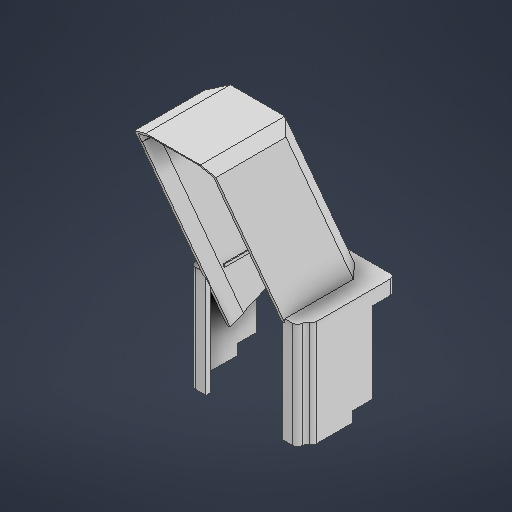
# Autodesk Inventor part: Event_Cover
Saved by Autodesk Inventor 2026 (Build 300175000, 175)
## iProperties
Created: 2025-07-07
Part Number: Event_Cover
Material: Generic
Document SubType Name: Modeling
Designer: Charl
Density: 1 g/cm^3
Appearance: Default
Author: Charl
Autodesk Inventor part; units mm, degrees
ref_plane "YZ Plane" through (0, 0, 0) normal (1, 0, 0) x (0, 1, 0)
ref_plane "XZ Plane" through (0, 0, 0) normal (0, 1, 0) x (-1, 0, 0)
sketch "Sketch1" plane through (0, 0, 0) normal (0, 1, 0) x (-1, 0, 0)
  line L0 (-58.5, -37.5625) -> (58.5, -37.5625)
  line L1 (58.5, -37.5625) -> (58.5, 37.5625)
  line L2 (58.5, 37.5625) -> (-58.5, 37.5625)
  line L3 (-58.5, 37.5625) -> (-58.5, -37.5625)
  line L4 (-58.5, -37.5625) -> (58.5, 37.5625) construction
  line L5 (58.5, -37.5625) -> (-58.5, 37.5625) construction
  line L6 (-61.5, 37.5625) -> (61.5, 37.5625)
  line L7 (61.5, 37.5625) -> (61.5, -40.5625)
  line L8 (61.5, -40.5625) -> (-61.5, -40.5625)
  line L9 (-61.5, -40.5625) -> (-61.5, 37.5625)
  line L10 (-38.5, 50.0625) -> (38.5, 50.0625)
  line L11 (38.5, 50.0625) -> (38.5, 25.0625)
  line L12 (38.5, 25.0625) -> (-38.5, 25.0625)
  line L13 (-38.5, 25.0625) -> (-38.5, 50.0625)
  line L14 (-38.5, 50.0625) -> (38.5, 25.0625) construction
  line L15 (38.5, 50.0625) -> (-38.5, 25.0625) construction
  line L16 (40, 37.5625) -> (40, 55.5625)
  line L17 (40, 55.5625) -> (55.75, 55.5625)
  line L18 (55.75, 55.5625) -> (55.75, 45.5625)
  line L19 (55.75, 45.5625) -> (61.5, 45.5625)
  line L20 (61.5, 45.5625) -> (61.5, 37.5625)
  line L21 (0, 358.9567) -> (0, -111.4305)
  line L22 (-40, 37.5625) -> (-40, 55.5625)
  line L23 (-40, 55.5625) -> (-55.75, 55.5625)
  line L24 (-55.75, 55.5625) -> (-55.75, 45.5625)
  line L25 (-55.75, 45.5625) -> (-61.5, 45.5625)
  line L26 (-61.5, 45.5625) -> (-61.5, 37.5625)
  circle A0 centre (0, 10.0625) radius 38.5
  line L27 (38.5, 25.0625) -> (-38.5, 25.0625)
  line L28 (-38.5, 25.0625) -> (-38.5, 10.0625)
  line L29 (-38.5, 10.0625) -> (38.5, 10.0625)
  line L30 (38.5, 10.0625) -> (38.5, 25.0625)
  point P0 (0, 0)
  point P1 (0, 37.5625)
  point P2 (-35.4577, 25.0625)
  point P3 (-38.5, 37.5625)
  point P4 (38.5, 37.5625)
  point P5 (35.4577, 25.0625)
  point P6 (38.5, 10.0625)
  dimension "d0" = 117
  dimension "d1" = 75.125
  dimension "d2" = 3
  dimension "d3" = 3
  dimension "d4" = 3
  dimension "d5" = 77
  dimension "d6" = 25
  dimension "d7" = 1.5
  dimension "d8" = 15.75
  dimension "d9" = 10
  dimension "d10" = 8
  dimension "d11" = 5.75
  dimension "d12" = 8
  dimension "d13" = 10
  dimension "d14" = 15.75
  dimension "d15" = 5.75
  dimension "d16" = 1.5
  dimension "d17" = 77
  dimension "d18" = 15
  dimension "d19" = 123
  dimension "d20" = 117
  dimension "d23" = 77
  constraints: 62 end point, 9 perpendicular, 8 parallel, 5 midpoint, 5 point on line, 5 symmetric about line, 3 horizontal, 1 centre point, 1 vertical
  measures "d0" distance of L2.end L1.end
  measures "d1" distance of L1.end L0.end
  measures "d2" distance between parallel lines of L1 L7
  measures "d3" distance between parallel lines of L9 L3
  measures "d4" distance between parallel lines of L8 L0
  measures "d5" distance of L11.end L12.end
  measures "d6" distance of L10.end L11.end
  measures "d7" distance from line of L11 L16.start
  measures "d8" distance of L16.end L17.end
  measures "d9" distance of L17.end L18.end
  measures "d10" distance of L19.end L6.end
  measures "d11" distance of L18.end L19.end
  measures "d12" distance of L26.start L6.start
  measures "d13" distance of L24.start L25.start
  measures "d14" distance of L23.start L24.start
  measures "d15" distance of L25.start L26.start
  measures "d16" distance between parallel lines of L13 L22
  measures "d17" diameter of A0
  measures "d18" distance from line of L12 A0.centre
  measures "d19" distance of L7.end L8.end
  measures "d20" distance of L0.start L0.end
  measures "d23" distance of L28.end L29.end
extrude "Extrusion2" add sketch "Sketch1" along normal blind 3 contours L3 L2 L13 L28 A0 L21 L0 | L0 L21 L8 L9 L6 L3 | L21 A0 L30 L11 L2 L1 L0 | L0 L1 L6 L7 L8 L21 | L6 L26 L25 L24 L23 L22 L2 | L2 L16 L17 L18 L19 L20 L6
sketch "Sketch3" plane through (0, 0, 0) normal (0, -1, 0) x (1, 0, 0)
  line L0 (-55.75, 55.5625) -> (-40, 55.5625) projected
  line L1 (-40, 55.5625) -> (-55.75, 55.5625)
  line L2 (-61.5, 45.5625) -> (-55.75, 45.5625) projected
  line L3 (-55.75, 55.5625) -> (-55.75, 45.5625)
  line L4 (-55.75, 45.5625) -> (-61.5, 45.5625)
  line L5 (-61.5, 45.5625) -> (-61.5, 20.5625)
  line L6 (-61.5, 20.5625) -> (-59.5, 20.5625)
  line L7 (-59.5, 20.5625) -> (-59.5, 43.5625)
  line L8 (-59.5, 43.5625) -> (-53.75, 43.5625)
  line L9 (-53.75, 43.5625) -> (-53.75, 50.5625)
  line L10 (-53.75, 50.5625) -> (-40, 50.5625)
  line L11 (-40, 55.5625) -> (-40, 37.5625) projected
  line L12 (-40, 55.5625) -> (-40, 50.5625)
  line L13 (55.75, 55.5625) -> (40, 55.5625)
  line L14 (40, 55.5625) -> (55.75, 55.5625)
  line L15 (61.5, 45.5625) -> (55.75, 45.5625)
  line L16 (55.75, 55.5625) -> (55.75, 45.5625)
  line L17 (55.75, 45.5625) -> (61.5, 45.5625)
  line L18 (61.5, 45.5625) -> (61.5, 20.5625)
  line L19 (61.5, 20.5625) -> (59.5, 20.5625)
  line L20 (59.5, 20.5625) -> (59.5, 43.5625)
  line L21 (59.5, 43.5625) -> (53.75, 43.5625)
  line L22 (53.75, 43.5625) -> (53.75, 50.5625)
  line L23 (53.75, 50.5625) -> (40, 50.5625)
  line L24 (40, 55.5625) -> (40, 37.5625)
  line L25 (40, 55.5625) -> (40, 50.5625)
  point P0 (0, 0)
  dimension "d31" = 5
  dimension "d32" = 2
  dimension "d33" = 2
  dimension "d34" = 25
  dimension "d35" = 2
  constraints: 46 end point, 7 perpendicular, 2 collinear, 2 point on line, 1 horizontal
  measures "d31" distance of L0.end L10.end
  measures "d32" distance between parallel lines of L3 L9
  measures "d33" distance between parallel lines of L2 L8
  measures "d34" distance between parallel lines of L6 L2
  measures "d35" distance between parallel lines of L5 L7
extrude "Extrusion3" add sketch "Sketch3" along normal blind 107.5
sketch "Sketch4" plane through (0, 0, 0) normal (0, -1, 0) x (1, 0, 0)
  line L0 (61.5, -40.5625) -> (-61.5, -40.5625)
  line L1 (61.5, -40.5625) -> (61.5, -16.5625)
  line L2 (61.5, -16.5625) -> (56, -16.5625)
  line L3 (56, -16.5625) -> (56, -37.5625)
  line L4 (56, -37.5625) -> (-56, -37.5625)
  line L5 (-56, -37.5625) -> (-56, -16.5625)
  line L6 (-56, -16.5625) -> (-61.5, -16.5625)
  line L7 (-61.5, -16.5625) -> (-61.5, -40.5625)
  line L8 (61.5, -17.0329) -> (61.5, 20.5625)
  line L9 (59.5, 43.5625) -> (59.5, 20.5625) projected
  line L10 (59.5, 20.5625) -> (59.5, -16.5625)
  line L11 (-61.5, 20.5625) -> (-59.5, 20.5625) projected
  line L12 (-59.5, 20.5625) -> (-59.5, -16.5625)
  line L13 (-61.5, -40.5625) -> (-61.5, 45.5625) projected
  line L14 (-61.5, 20.5625) -> (-61.5, -16.5625)
  line L15 (61.5, 20.5625) -> (61.5, 45.5625) projected
  line L16 (61.5, 20.5625) -> (59.5, 20.5625)
  line L17 (-59.5, 20.5625) -> (-61.5, 20.5625)
  point P0 (0, 0)
  dimension "d38" = 24
  dimension "d39" = 24
  dimension "d40" = 5.5
  dimension "d41" = 5.5
  dimension "d42" = 3
  dimension "d43" = 2
  dimension "d44" = 2
  constraints: 28 end point, 6 perpendicular, 4 point on line, 3 horizontal, 3 vertical, 1 collinear
  measures "d38" distance between parallel lines of L0 L6
  measures "d39" distance of L0.start L1.end
  measures "d40" distance of L1.end L2.end
  measures "d41" distance of L5.end L6.end
  measures "d42" distance between parallel lines of L0 L4
  measures "d43" distance between parallel lines of L8 L10
  measures "d44" distance between parallel lines of L13 L12
extrude "Extrusion4" add sketch "Sketch4" along normal blind 12
fillet "Fillet1" radius 5 16 edges at (-55.75, -52.25, 55.5625) (-55.75, -52.25, 45.5625) (-61.5, -52.25, 45.5625) (-61.5, -4.5, -40.5625) (61.5, -4.5, -40.5625) (55.75, -52.25, 45.5625) (55.75, -52.25, 55.5625) (61.5, -52.25, 45.5625) (53.75, -53.75, 50.5625) (59.5, -53.75, 43.5625) (53.75, -53.75, 43.5625) (-53.75, -53.75, 50.5625) (-53.75, -53.75, 43.5625) (-59.5, -53.75, 43.5625) (56, -6, -37.5625) (-56, -6, -37.5625)
chamfer "Chamfer1" distance 3.5 angle 45 2 edges at (56, -6, -16.5625) (-56, -6, -16.5625)
ref_plane "Work Plane1" through (-55.75, 3, 55.5625) normal (0, 0.9187912, 0.3947439) x (1, 0, 0)
sketch "Sketch5" plane through (-55.75, 3, 55.5625) normal (0, 0.9187912, 0.3947439) x (1, 0, 0)
  line L0 (16.25, 24.0537) -> (16.25, 75.6785)
  line L1 (16.25, 75.6785) -> (95.25, 75.6785)
  line L2 (95.25, 75.6785) -> (95.25, 24.0537)
  line L3 (55.75, 49.8661) -> (16.25, 75.6785) construction
  line L4 (55.75, 49.8661) -> (95.25, 75.6785) construction
  line L5 (13.25, 20.0537) -> (13.25, 79.6785)
  line L6 (13.25, 79.6785) -> (98.25, 79.6785)
  line L7 (98.25, 79.6785) -> (98.25, 20.0537)
  line L8 (55.75, 49.8661) -> (98.25, 79.6785) construction
  ellipse E0 centre (55.75, 40.6208) end of major axis (94.25, 40.6208) minor radius 35.3735 (94.25, 40.6208) -> (17.25, 40.6208) ccw projected
  ellipse E1 centre (55.75, 41.805) end of major axis (94.25, 41.805) minor radius 35.3735 (94.25, 41.805) -> (17.25, 41.805) ccw projected
  line L9 (5, 0) -> (15.75, 0) construction
  line L10 (-163.9514, 0) -> (184.7014, 0) construction
  line L11 (13.25, 20.0537) -> (13.25, -1.5)
  line L12 (13.25, -1.5) -> (16.75, -1.5)
  line L13 (16.75, -1.5) -> (16.75, 13.3942)
  line L14 (16.75, 13.3942) -> (16.25, 13.3942)
  line L15 (16.25, 13.3942) -> (16.25, 20.0537)
  line L16 (55.75, 49.8661) -> (13.25, 79.6785) construction
  line L17 (16.25, 24.0537) -> (16.25, 20.0537)
  line L18 (17.25, 15.354) -> (17.25, 40.6208) projected
  line L19 (55.75, 112.6041) -> (55.75, -12.8719)
  line L20 (55.75, 112.6041) -> (181.2261, 112.6041) construction
  line L21 (95.25, 24.0537) -> (95.25, 75.6785)
  line L22 (98.25, 20.0537) -> (98.25, 79.6785)
  line L23 (106.5, 0) -> (95.75, 0) construction
  line L24 (98.25, 20.0537) -> (98.25, -1.5)
  line L25 (98.25, -1.5) -> (94.75, -1.5)
  line L26 (94.75, -1.5) -> (94.75, 13.3942)
  line L27 (94.75, 13.3942) -> (95.25, 13.3942)
  line L28 (95.25, 13.3942) -> (95.25, 20.0537)
  line L29 (95.25, 24.0537) -> (95.25, 20.0537)
  arc A0 (94.25, 40.6208) -> (66.3648, 75.6785) centre (55.7096, 38.5843) ccw
  arc A1 (45.0543, 75.6785) -> (17.25, 41.805) centre (55.7096, 38.5843) ccw
  point P0 (55.75, 49.8661)
  point P1 (55.75, 77.1785)
  point P2 (10.375, 0)
  point P3 (101.125, 0)
  point P4 (94.25, 15.354)
  dimension "d52" = 79
  dimension "d53" = 4
  dimension "d54" = 3
  dimension "d56" = 27.3124
  dimension "d57" = 1.5
  dimension "d58" = 1.5
  dimension "d59" = 3.5
  dimension "d60" = 90
  constraints: 56 end point, 8 point on line, 8 symmetric about line, 4 point on circle, 3 horizontal, 3 midpoint, 3 parallel, 2 centre point, 2 vertical, 1 perpendicular, 3 other
  measures "d52" distance of L0.end L1.end
  measures "d53" distance between parallel lines of L1 L6
  measures "d54" distance between parallel lines of L0 L5
  measures "d56" distance of point (55.75, 49.866) point (55.75, 77.178)
  measures "d57" distance from line of point (55.75, 77.178) L1
  measures "d58" distance from line of L11.end L10
  measures "d59" distance of L11.end L12.end
  measures "d60" angle of L19 L20
extrude "Extrusion5" add sketch "Sketch5" along normal blind 150 and the other way blind 65.325 contours L17 L15 L14 L13 L12 L11 L5 L6 L19 E1 L1 L0 | E1 L19 E0 L1 | L19 L6 L7 L24 L25 L26 L27 L28 L29 L2 L1 E1 | E1 L1 E0 L19 | E0 L19 L1 | E0 L1 L19
chamfer "Chamfer2" distance 14 angle 45 4 edges at (-39.5, 86.8461, 9.2182) (-42.5, 87.6356, 5.2039) (42.5, 87.6356, 5.2039) (39.5, 86.8461, 9.2182)
sketch "Sketch6" plane through (0, -12, 0) normal (0, -1, 0) x (1, 0, 0)
  line L0 (-59.5, 38.5625) -> (-59.5, -16.5625) projected
  line L1 (-59.5, -16.5625) -> (-59.5, 20.5625)
  line L2 (-61.5, 41.5106) -> (-61.5, 20.5625) projected
  line L3 (-59.5, 20.5625) -> (-61.5, 20.5625)
  line L4 (-61.5, 20.5625) -> (-61.5, -16.5625)
  line L5 (-61.5, -16.5625) -> (-59.5, -16.5625)
  line L6 (0, -16.4612) -> (0, 16.4612)
  line L7 (59.5, -16.5625) -> (59.5, 20.5625)
  line L8 (59.5, 20.5625) -> (61.5, 20.5625)
  line L9 (61.5, 20.5625) -> (61.5, -16.5625)
  line L10 (61.5, -16.5625) -> (59.5, -16.5625)
  point P0 (0, 0)
  constraints: 18 end point, 4 symmetric about line, 2 perpendicular, 1 horizontal, 1 midpoint, 1 point on line, 1 vertical
extrude "Extrusion6" add sketch "Sketch6" along normal blind 95.5
sketch "Sketch7" plane through (0, -107.5, 0) normal (0, -1, 0) x (1, 0, 0)
  line L0 (59.5, 38.5625) -> (59.5, -16.5625) projected
  line L1 (59.5, -16.5625) -> (59.5, 3.4375)
  line L2 (59.5, 3.4375) -> (61.5, 3.4375)
  line L3 (61.5, -16.5625) -> (61.5, 41.5106) projected
  line L4 (61.5, 3.4375) -> (61.5, -16.5625)
  line L5 (59.5, -16.5625) -> (61.5, -16.5625)
  line L6 (0, 21.9303) -> (0, -27.0854)
  line L7 (-59.5, -16.5625) -> (-59.5, 3.4375)
  line L8 (-59.5, 3.4375) -> (-61.5, 3.4375)
  line L9 (-61.5, 3.4375) -> (-61.5, -16.5625)
  line L10 (-59.5, -16.5625) -> (-61.5, -16.5625)
  point P0 (0, 0)
  dimension "d70" = 20
  constraints: 18 end point, 4 symmetric about line, 2 perpendicular, 2 point on line, 2 vertical
  measures "d70" distance of L0.end L1.end
extrude "Extrusion7" cut sketch "Sketch7" against normal blind 11
ref_plane "Work Plane4" through (-39.5, 155.6359, 80.286) normal (0, 0, 1) x (1, 0, 0)
sketch "Sketch16" plane through (-39.5, 155.6359, 80.286) normal (0, 0, 1) x (1, 0, 0)
  line L0 (-3, -152.6359) -> (-3, 11.1089) projected
  line L1 (-3, 11.1089) -> (-3, -23.8911)
  line L2 (-3, 11.1089) -> (32, 11.1089) construction
  line L3 (82, 11.1089) -> (82, -152.6359) projected
  line L4 (82, 11.1089) -> (82, -76.5693)
  line L5 (68, 16.6354) -> (11, 16.6354) projected
  line L6 (-3, 11.1089) -> (11, 16.6354)
  line L7 (11, 16.6354) -> (68, 16.6354)
  line L8 (68, 16.6354) -> (82, 11.1089)
  line L9 (0, 9.53) -> (0, -152.6359) projected
  line L10 (0, 9.53) -> (0, -23.8911)
  line L11 (14, -152.6359) -> (14, 15.0564) projected
  line L12 (0, 9.53) -> (14, 15.0564)
  line L13 (79, 9.53) -> (65, 15.0564) projected
  line L14 (14, 15.0564) -> (65, 15.0564)
  line L15 (79, -152.6359) -> (79, 9.53) projected
  line L16 (65, 15.0564) -> (79, 9.53)
  line L17 (79, 9.53) -> (79, -76.5693)
  line L18 (-3, -23.8911) -> (0, -23.8911)
  line L19 (79, -76.5693) -> (82, -76.5693)
  point P0 (39.5, -155.6359)
  point P1 (-3, -23.8911)
  dimension "d90" = 35
  dimension "d91" = 90
  dimension "d92" = 100
  constraints: 26 end point, 4 perpendicular, 3 point on line, 2 collinear, 1 horizontal
  measures "d90" distance of L0.end L1.end
  measures "d91" angle of L1 L2
  measures "d92" distance of L1.end L4.end
extrude "Extrusion12" add sketch "Sketch16" against normal through all
sketch "Sketch17" plane through (-39.5, 155.6359, 80.286) normal (0, 0, 1) x (1, 0, 0)
  line L0 (0, 0) -> (-3, 0) projected
  line L1 (-3, -152.6359) -> (-3, 11.1089) projected
  line L2 (-3, 0) -> (-3, 11.1089)
  line L3 (-3, 11.1089) -> (11, 16.6354) projected
  line L4 (-3, 11.1089) -> (11, 16.6354)
  line L5 (82, 11.1089) -> (68, 16.6354) projected
  line L6 (11, 16.6354) -> (68, 16.6354)
  line L7 (82, 0) -> (79, 0) projected
  line L8 (82, 11.1089) -> (82, 0)
  line L9 (82, 0) -> (79, 0)
  line L10 (79, 9.53) -> (65, 15.0564) projected
  line L11 (79, 0) -> (79, 9.53)
  line L12 (14, 15.0564) -> (65, 15.0564) projected
  line L13 (79, 9.53) -> (65, 15.0564)
  line L14 (65, 15.0564) -> (14, 15.0564)
  line L15 (0, 9.53) -> (0, -152.6359) projected
  line L16 (14, 15.0564) -> (0, 9.53)
  line L17 (0, 9.53) -> (0, 0)
  point P0 (39.5, -155.6359)
  constraints: 20 end point, 3 collinear, 2 perpendicular, 2 vertical, 1 parallel
extrude "Extrusion13" add sketch "Sketch17" along normal up to surface surface through (39, 2.4079, 56.9407) normal (0, -0.3947439, 0.9187912)
sketch "Sketch18" plane through (-55.75, 140.8187, 114.7741) normal (0, 0.9187912, 0.3947439) x (1, 0, 0)
  line L0 (13.25, 37.5363) -> (13.25, -1.5) projected
  line L1 (13.25, -1.5) -> (16.75, -1.5) projected
  line L2 (13.25, 37.5363) -> (13.25, -1.5)
  line L3 (16.75, -1.5) -> (16.75, 13.3942) projected
  line L4 (13.25, -1.5) -> (16.75, -1.5)
  line L5 (16.75, -1.5) -> (16.75, 13.3942)
  line L6 (16.25, 13.3942) -> (16.25, 37.5363) projected
  line L7 (16.75, 13.3942) -> (16.25, 13.3942)
  line L8 (16.25, 13.3942) -> (16.25, 37.5363)
  line L9 (16.25, 37.5363) -> (13.25, 37.5363) projected
  line L10 (16.25, 37.5363) -> (13.25, 37.5363)
  line L11 (98.25, -1.5) -> (98.25, 37.5363) projected
  line L12 (94.75, -1.5) -> (98.25, -1.5) projected
  line L13 (98.25, 37.5363) -> (98.25, -1.5)
  line L14 (95.25, 13.3942) -> (94.75, 13.3942) projected
  line L15 (95.25, 37.6402) -> (95.25, 13.3942)
  line L16 (94.75, 13.3942) -> (94.75, -1.5) projected
  line L17 (95.25, 13.3942) -> (94.75, 13.3942)
  line L18 (94.75, 13.3942) -> (94.75, -1.5)
  line L19 (94.75, -1.5) -> (98.25, -1.5)
  line L20 (98.25, 37.5363) -> (95.25, 37.5363) projected
  line L21 (95.25, 37.6402) -> (98.25, 37.5363)
  point P0 (55.75, 49.8661)
  constraints: 24 end point, 6 perpendicular, 3 collinear, 2 vertical
extrude "Extrusion14" add sketch "Sketch18" along normal up to surface contours L9 L6 L7 L3 L1 L0 | L12 L16 L14 L15 L20 L11 surface through (39.5, 155.6359, 80.286) normal (0, -1, 0)
equation "\"d3\" = d2"
equation "\"d4\" = d2"
equation "\"d7\" = 0.5 * d2"
equation "\"d12\" = d10"
equation "\"d38\" = d39"
equation "\"d41\" = d40"
body "Solid2"
